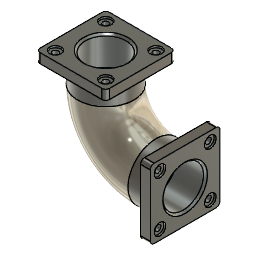
MARS_4 (Autodesk Fusion 360 design; units mm, degrees)
part number: 2026-05-31-13-26-19-711
Autodesk Fusion 360 part; units mm, degrees
sketch "Sketch1" plane through (0, 0, 0) normal (0, 1, 0) x (1, 0, 0)
  line L0 (0, 0) -> (0, 150)
  line L1 (260, 410) -> (410, 410)
  arc A0 (260, 410) -> (0, 150) centre (260, 150) ccw
  point P0 (0, 410)
  dimension "d1" = 410
  dimension "d2" = 410
  dimension "d3" = 260
  constraint coincident L0.start origin
  constraint vertical L0
  constraint perpendicular L0 L1
  constraint coincident P0 L1
  constraint coincident P0 L0
  constraint tangent L1 A0
  constraint tangent L0 A0
  measures "d1" distance of L0.start P0
  measures "d2" distance of P0 L1.end
  measures "d3" radius of A0
sketch "Sketch2" plane through (0, 0, 0) normal (0, 0, 1) x (1, 0, 0)
  circle A0 centre (0, 0) radius 145
  circle A1 centre (0, 0) radius 105
  dimension "d4" = 290
  dimension "d5" = 210
  constraint coincident A0.centre A1.centre
  constraint concentric A0 A1
  measures "d4" diameter of A0
  measures "d5" diameter of A1
sweep "Sweep1" add profiles "Sketch2" path "Sketch1" along L1 A0 L0 section 1
sketch "Sketch3" plane through (0, 0, 0) normal (0, 0, 1) x (-1, 0, 0)
  circle A0 centre (0, 0) radius 105
  circle A1 centre (0, 0) radius 145
  line L0 (-180, 180) -> (180, 180)
  line L1 (180, 180) -> (180, -180)
  line L2 (180, -180) -> (-180, -180)
  line L3 (-180, -180) -> (-180, 180)
  line L4 (-180, 180) -> (180, -180) construction
  line L5 (180, 180) -> (-180, -180) construction
  dimension "d12" = 360
  dimension "d13" = 360
  constraint horizontal L0
  constraint perpendicular L0 L1
  constraint parallel L0 L2
  constraint parallel L1 L3
  constraint coincident L4 A0.centre
  constraint coincident L5 A0.centre
  constraint coincident A0.centre A1.centre
  measures "d12" distance of L1.end L2.end
  measures "d13" distance of L0.end L1.end
extrude "Extrude1" add sketch "Sketch3" against normal blind 50 contours L0 L1 L2 L3
sketch "Sketch4" plane through (410, 0, 0) normal (1, 0, 0) x (0, 1, 0)
  circle A0 centre (0, -410) radius 105
  circle A1 centre (0, -410) radius 145
  line L0 (180, -580) -> (-180, -580)
  line L1 (-180, -580) -> (-180, -220)
  line L2 (-180, -220) -> (180, -220)
  line L3 (180, -220) -> (180, -580)
  line L4 (180, -580) -> (-180, -220) construction
  line L5 (-180, -580) -> (180, -220) construction
  point P0 (0, -400)
  dimension "d16" = 360
  dimension "d17" = 360
  constraint horizontal L0
  constraint perpendicular L0 L1
  constraint parallel L0 L2
  constraint parallel L1 L3
  constraint coincident L4 P0
  constraint coincident L5 P0
  measures "d16" distance of L1.end L2.end
  measures "d17" distance of L0.end L1.end
extrude "Extrude2" add sketch "Sketch4" against normal blind 50 contours L0 L1 L2 L3
fillet "Fillet1" radius 20 4 edges at (180, -180, -25) (180, 180, -25) (-180, -180, -25) (-180, 180, -25)
fillet "Fillet2" radius 20 4 edges at (385, -180, -220) (385, 180, -220) (385, 180, -580) (385, -180, -580)
fillet "Fillet3" radius 10 2 edges at (-135.1875, 52.4342, -50) (360, -52.4342, -545.1875)
sketch "Sketch5" plane through (0, 0, 0) normal (0, 0, 1) x (-1, 0, 0)
  arc A0 (160, -180) -> (180, -160) centre (160, -160) ccw
  line L0 (180, -160) -> (180, 160)
  arc A1 (180, 160) -> (160, 180) centre (160, 160) ccw
  line L1 (160, 180) -> (-160, 180)
  arc A2 (-160, 180) -> (-180, 160) centre (-160, 160) ccw
  line L2 (-180, 160) -> (-180, -160)
  arc A3 (-180, -160) -> (-160, -180) centre (-160, -160) ccw
  line L3 (-160, -180) -> (160, -180)
  circle A4 centre (0, 0) radius 105
  line L4 (130, 130) -> (-130, 130) construction
  line L5 (-130, 130) -> (-130, -130) construction
  line L6 (-130, -130) -> (130, -130) construction
  line L7 (130, -130) -> (130, 130) construction
  line L8 (130, 130) -> (-130, -130) construction
  line L9 (-130, 130) -> (130, -130) construction
  dimension "d26" = 260
  dimension "d27" = 260
  constraint horizontal L4
  constraint perpendicular L4 L5
  constraint parallel L4 L6
  constraint parallel L5 L7
  constraint coincident L8 A4.centre
  constraint coincident L9 A4.centre
  constraint coincident A4.centre origin
  measures "d26" distance of L5.end L6.end
  measures "d27" distance of L4.end L5.end
hole "Hole1" at (130, 130, 0) at (-130, 130, 0) at (-130, -130, 0) at (130, -130, 0) direction (0, 0, -1) diameter 30 depth 50 tip angle 180 counterbore diameter 60 counterbore depth 10
sketch "Sketch6" plane through (410, 0, 0) normal (1, 0, 0) x (0, 1, 0)
  arc A0 (-180, -560) -> (-160, -580) centre (-160, -560) ccw
  line L0 (-160, -580) -> (160, -580)
  arc A1 (160, -580) -> (180, -560) centre (160, -560) ccw
  line L1 (180, -560) -> (180, -240)
  arc A2 (180, -240) -> (160, -220) centre (160, -240) ccw
  line L2 (160, -220) -> (-160, -220)
  arc A3 (-160, -220) -> (-180, -240) centre (-160, -240) ccw
  line L3 (-180, -240) -> (-180, -560)
  circle A4 centre (0, -410) radius 105
sketch "Sketch7" plane through (410, 0, 0) normal (1, 0, 0) x (0, 1, 0)
  line L0 (130, -270) -> (-130, -270) construction
  line L1 (-130, -270) -> (-130, -530) construction
  line L2 (-130, -530) -> (130, -530) construction
  line L3 (130, -530) -> (130, -270) construction
  line L4 (130, -270) -> (-130, -530) construction
  line L5 (-130, -270) -> (130, -530) construction
  point P0 (0, -400)
  dimension "d33" = 260
  dimension "d34" = 260
  constraint horizontal L0
  constraint perpendicular L0 L1
  constraint parallel L0 L2
  constraint parallel L1 L3
  constraint coincident L4 P0
  constraint coincident L5 P0
  measures "d33" distance of L1.end L2.end
  measures "d34" distance of L0.end L1.end
hole "Hole2" at (410, 130, -270) at (410, -130, -270) at (410, -130, -530) at (410, 130, -530) direction (-1, 0, 0) diameter 30 depth 50 tip angle 180 counterbore diameter 60 counterbore depth 10
chamfer "Chamfer1" distance 10 angle 45 2 edges at (410, -37.9696, -507.8944) (-97.8944, 37.9696, 0)
sketch "Sketch8" plane through (0, 0, 0) normal (0, 0, 1) x (-1, 0, 0)
  circle A0 centre (130, 130) radius 30
  circle A1 centre (-130, -130) radius 30
  circle A2 centre (130, -130) radius 30
  circle A3 centre (-130, 130) radius 30
  arc A4 (160, -180) -> (180, -160) centre (160, -160) ccw
  line L0 (180, -160) -> (180, 160)
  arc A5 (180, 160) -> (160, 180) centre (160, 160) ccw
  line L1 (160, 180) -> (-160, 180)
  arc A6 (-160, 180) -> (-180, 160) centre (-160, 160) ccw
  line L2 (-180, 160) -> (-180, -160)
  arc A7 (-180, -160) -> (-160, -180) centre (-160, -160) ccw
  line L3 (-160, -180) -> (160, -180)
  circle A8 centre (0, 0) radius 115
sketch "Sketch9" plane through (410, 0, 0) normal (1, 0, 0) x (0, 1, 0)
sketch "Sketch10" plane through (0, 0, 0) normal (0, 0, 1) x (-1, 0, 0)
